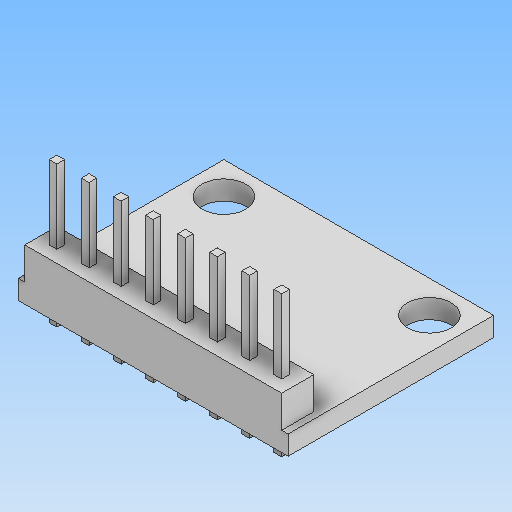
# Autodesk Inventor part: 10_MPU_6050
Saved by Autodesk Inventor 2020 (Build 240168000, 168)
## iProperties
Created: 2019-10-15
Part Number: 10_MPU_6050
Material: Generico
Document SubType Name: Modeling
Designer: socci
Density: 1 g/cm^3
Appearance: Default
Author: socci
Autodesk Inventor part; units mm, degrees
ref_plane "YZ Plane" through (0, 0, 0) normal (1, 0, 0) x (0, 1, 0)
ref_plane "XZ Plane" through (0, 0, 0) normal (0, 1, 0) x (-1, 0, 0)
ref_plane "XY Plane" through (0, 0, 0) normal (0, 0, 1) x (1, 0, 0)
sketch "Schizzo1" plane through (0, 0, 0) normal (0, 1, 0) x (-1, 0, 0)
  line L0 (10.5, 8) -> (-10.5, 8)
  line L1 (-10.5, 8) -> (-10.5, -8)
  line L2 (-10.5, -8) -> (10.5, -8)
  line L3 (10.5, -8) -> (10.5, 8)
  line L4 (10.5, 8) -> (-10.5, -8) construction
  line L5 (-10.5, 8) -> (10.5, -8) construction
  point P0 (0, 0)
  point P1 (0, 0)
  point P2 (0, 0)
  dimension "d0" = 16
  dimension "d1" = 21
  constraints: 12 end point, 3 midpoint, 2 parallel, 1 coincident, 1 horizontal, 1 perpendicular
  measures "d0" distance of L0.end L1.end
  measures "d1" distance of L0.start L0.end
extrude "Estrusione1" add sketch "Schizzo1" along normal blind 1.5
sketch "Schizzo2" plane through (0, 1.5, 0) normal (0, 1, 0) x (1, 0, 0)
  line L0 (10.5, 8) -> (-10.5, 8) projected
  line L1 (-10.5, 8) -> (-8, 8)
  line L2 (-8, 8) -> (-8, 5.5)
  line L3 (10.5, 8) -> (8, 8)
  line L4 (8, 8) -> (8, 5.5)
  point P0 (0, 0)
  dimension "d16" = 2.5
  dimension "d17" = 2.5
  dimension "d18" = 2.5
  dimension "d19" = 2.5
  constraints: 8 end point, 2 perpendicular, 2 point on line
  measures "d16" distance of L0.end L1.end
  measures "d17" distance of L1.end L2.end
  measures "d18" distance of L0.start L3.end
  measures "d19" distance of L3.end L4.end
hole "Foro1" at (-8, 1.5, -5.5) at (8, 1.5, -5.5) direction (0, -1, 0) diameter 3.4 depth 1.5 tip angle 118 clearance for "Vite a testa esagonale" size "M3" standard "ANSI - Profilo M Metrico"
sketch "Schizzo4" plane through (0, 1.5, 0) normal (0, 1, 0) x (1, 0, 0)
  line L0 (10, -5.5) -> (-10, -5.5)
  line L1 (-10, -5.5) -> (-10, -8)
  line L2 (-10, -8) -> (10, -8)
  line L3 (10, -8) -> (10, -5.5)
  line L4 (10, -5.5) -> (-10, -8) construction
  line L5 (-10, -5.5) -> (10, -8) construction
  line L6 (-10.5, -8) -> (10.5, -8) projected
  point P0 (0, 0)
  point P1 (0, -6.75)
  point P2 (0, -8)
  dimension "d45" = 20
  dimension "d46" = 2.5
  constraints: 12 end point, 4 midpoint, 2 parallel, 1 horizontal, 1 perpendicular
  measures "d45" distance of L0.start L0.end
  measures "d46" distance of L0.end L1.end
extrude "Estrusione2" add sketch "Schizzo4" along normal blind 2.5
sketch "Schizzo6" plane through (0, 4, 0) normal (0, 1, 0) x (1, 0, 0)
  line L0 (-8.75, -6.75) -> (-6.25, -6.75)
  line L1 (-9.05, -7.05) -> (-9.05, -6.45)
  line L2 (-9.05, -6.45) -> (-8.45, -6.45)
  line L3 (-8.45, -6.45) -> (-8.45, -7.05)
  line L4 (-8.45, -7.05) -> (-9.05, -7.05)
  line L5 (-6.25, -6.75) -> (-3.75, -6.75)
  line L6 (-6.55, -7.05) -> (-6.55, -6.45)
  line L7 (-6.55, -6.45) -> (-5.95, -6.45)
  line L8 (-5.95, -6.45) -> (-5.95, -7.05)
  line L9 (-5.95, -7.05) -> (-6.55, -7.05)
  line L10 (-3.75, -6.75) -> (-1.25, -6.75)
  line L11 (-4.05, -7.05) -> (-4.05, -6.45)
  line L12 (-4.05, -6.45) -> (-3.45, -6.45)
  line L13 (-3.45, -6.45) -> (-3.45, -7.05)
  line L14 (-3.45, -7.05) -> (-4.05, -7.05)
  line L15 (-1.25, -6.75) -> (1.25, -6.75)
  line L16 (-1.55, -7.05) -> (-1.55, -6.45)
  line L17 (-1.55, -6.45) -> (-0.95, -6.45)
  line L18 (-0.95, -6.45) -> (-0.95, -7.05)
  line L19 (-0.95, -7.05) -> (-1.55, -7.05)
  line L20 (1.25, -6.75) -> (3.75, -6.75)
  line L21 (0.95, -7.05) -> (0.95, -6.45)
  line L22 (0.95, -6.45) -> (1.55, -6.45)
  line L23 (1.55, -6.45) -> (1.55, -7.05)
  line L24 (1.55, -7.05) -> (0.95, -7.05)
  line L25 (3.75, -6.75) -> (6.25, -6.75)
  line L26 (3.45, -7.05) -> (3.45, -6.45)
  line L27 (3.45, -6.45) -> (4.05, -6.45)
  line L28 (4.05, -6.45) -> (4.05, -7.05)
  line L29 (4.05, -7.05) -> (3.45, -7.05)
  line L30 (6.25, -6.75) -> (8.75, -6.75)
  line L31 (5.95, -7.05) -> (5.95, -6.45)
  line L32 (5.95, -6.45) -> (6.55, -6.45)
  line L33 (6.55, -6.45) -> (6.55, -7.05)
  line L34 (6.55, -7.05) -> (5.95, -7.05)
  line L35 (8.45, -7.05) -> (8.45, -6.45)
  line L36 (8.45, -6.45) -> (9.05, -6.45)
  line L37 (9.05, -6.45) -> (9.05, -7.05)
  line L38 (9.05, -7.05) -> (8.45, -7.05)
  line L39 (-8.75, -6.75) -> (-10, -6.75)
  line L40 (-10, -8) -> (10, -8) projected
  line L41 (-10, -8) -> (-10, -6.75)
  line L42 (-10, -8) -> (-8.75, -8) construction
  point P0 (0, 0)
  dimension "d47" = 2.5
  dimension "d48" = 0.6
  dimension "d49" = 2.5
  dimension "d50" = 0.6
  dimension "d51" = 2.5
  dimension "d52" = 0.6
  dimension "d53" = 2.5
  dimension "d54" = 0.6
  dimension "d55" = 2.5
  dimension "d56" = 0.6
  dimension "d57" = 2.5
  dimension "d58" = 0.6
  dimension "d59" = 2.5
  dimension "d60" = 0.6
  dimension "d62" = 0.6
  dimension "d63" = 1.25
  dimension "d64" = 1.25
  dimension "d65" = 90
  constraints: 84 end point, 9 horizontal, 7 coincident, 1 perpendicular, 1 vertical, 72 other
  measures "d47" distance of L0.start L0.end
  measures "d48" distance of L1.start L3.end
  measures "d49" distance of L5.start L5.end
  measures "d50" distance of L6.start L8.end
  measures "d51" distance of L10.start L10.end
  measures "d52" distance of L11.start L13.end
  measures "d53" distance of L15.start L15.end
  measures "d54" distance of L16.start L18.end
  measures "d55" distance of L20.start L20.end
  measures "d56" distance of L21.start L23.end
  measures "d57" distance of L25.start L25.end
  measures "d58" distance of L26.start L28.end
  measures "d59" distance of L30.start L30.end
  measures "d60" distance of L31.start L33.end
  measures "d62" distance of L35.start L37.end
  measures "d63" distance of L39.start L39.end
  measures "d64" distance of L40.start L41.end
  measures "d65" angle of L42 L41
extrude "Estrusione3" add sketch "Schizzo6" along normal blind 5.75 and the other way blind 5.25
